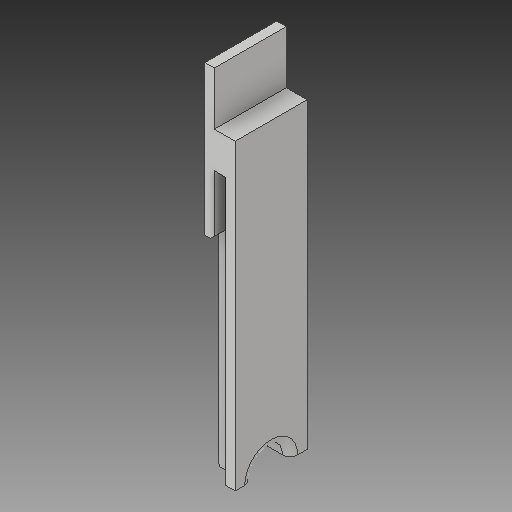
# Autodesk Inventor part: BOttom Clip
Saved by Autodesk Inventor 2017 (Build 210142000, 142)
## iProperties
Created: 2018-02-13
Part Number: BOttom Clip
Material: Generic
Document SubType Name: Modeling
Designer: Arjuna
Density: 1 g/cm^3
Appearance: Default
Author: Arjuna
Autodesk Inventor part; units mm, degrees
ref_plane "YZ Plane" through (0, 0, 0) normal (1, 0, 0) x (0, 1, 0)
ref_plane "XZ Plane" through (0, 0, 0) normal (0, 1, 0) x (-1, 0, 0)
ref_plane "XY Plane" through (0, 0, 0) normal (0, 0, 1) x (1, 0, 0)
sketch "Sketch1" plane through (0, 0, 0) normal (1, 0, 0) x (0, 1, 0)
  line L0 (40, 9.5) -> (-40, 9.5)
  line L1 (-40, 9.5) -> (-40, -9.5)
  line L2 (-40, -9.5) -> (40, -9.5)
  line L3 (40, -9.5) -> (40, 9.5)
  point P0 (0, 0)
  dimension "d0" = 19
  dimension "d1" = 80
  dimension "d2" = 9.5
  dimension "d3" = 40
  constraints: 8 end point, 2 parallel, 1 horizontal, 1 perpendicular
  measures "d0" distance between parallel lines of L2 L0
  measures "d1" distance between parallel lines of L1 L3
  measures "d2" distance from line of L0 point (0, 0)
  measures "d3" distance from line of point (0, 0) L3
extrude "Extrusion1" add sketch "Sketch1" along normal blind 8
sketch "Sketch2" plane through (0, 40, 9.5) normal (0, 1, 0) x (1, 0, 0)
  line L0 (0, 19) -> (0, 0) projected
  line L1 (0, 0) -> (8, 0) projected
  line L2 (8, 19) -> (8, 0) projected
  line L3 (0, 19) -> (8, 19) projected
  line L4 (0, 0) -> (2.5, 0)
  line L5 (2.5, 0) -> (2.5, 19)
  line L6 (2.5, 19) -> (0, 19)
  line L7 (0, 19) -> (0, 0)
  point P0 (0, 9.5)
  dimension "d6" = 2.5
  constraints: 8 end point, 2 parallel, 1 horizontal, 1 perpendicular, 1 point on line
  measures "d6" distance of L6.end L5.end
extrude "Extrusion2" add sketch "Sketch2" along normal blind 14 contours L3 L5 L1 L0
sketch "Sketch4" plane through (8, -40, -9.5) normal (0, 0, -1) x (-1, 0, 0)
  line L0 (8, 0) -> (8, 94) projected
  line L1 (5.5, 94) -> (8, 94) projected
  line L2 (5.5, 80) -> (5.5, 94) projected
  line L3 (5.5, 80) -> (0, 80) projected
  line L4 (0, 0) -> (0, 80) projected
  line L5 (8, 0) -> (0, 0) projected
  line L6 (2.5, 70.5) -> (5.5, 70.5)
  line L7 (5.5, 70.5) -> (5.5, 54.5)
  line L8 (5.5, 54.5) -> (2.5, 54.5)
  line L9 (2.5, 54.5) -> (2.5, 70.5)
  line L10 (2.5, 54.5) -> (8, 54.5)
  line L11 (8, 54.5) -> (8, 0)
  line L12 (8, 0) -> (2.5, 0)
  line L13 (2.5, 0) -> (2.5, 54.5)
  point P0 (8, 40)
  dimension "d9" = 3
  dimension "d10" = 9.5
  dimension "d11" = 16
  dimension "d12" = 2.5
  dimension "d13" = 2.5
  constraints: 16 end point, 4 parallel, 2 horizontal, 2 perpendicular
  measures "d9" distance of L7.end L8.end
  measures "d10" distance between parallel lines of L6 L3
  measures "d11" distance between parallel lines of L8 L6
  measures "d12" distance between parallel lines of L9 L4
  measures "d13" distance between parallel lines of L0 L7
extrude "Extrusion3" cut sketch "Sketch4" against normal blind 3.5 contours L5 L13 L8 L10 L0 | L8 L9 L6 L7
mirror "Mirror1" about plane through (0, 0, 0) normal (0, 0, 1) of "Extrusion3"
chamfer "Chamfer1" distance 1 angle 45 2 edges at (2.5, 14.5, 7.75) (2.5, 14.5, -7.75)
sketch "Sketch5" plane through (8, 0, 0) normal (1, 0, 0) x (0, 0, -1)
  line L0 (-9.5, 40) -> (-9.5, -40) projected
  line L1 (-9.5, -40) -> (9.5, -40) projected
  line L2 (9.5, -40) -> (9.5, 40) projected
  line L3 (9.5, 40) -> (-9.5, 40) projected
  circle A0 centre (0, -40) radius 5
  point P0 (0, 0)
  dimension "d19" = 10
  constraints: 1 centre point, 1 midpoint
  measures "d19" diameter of A0
extrude "Extrusion4" cut sketch "Sketch5" against normal through all contours A0 L1 | L1 A0
fillet "Fillet1" radius 2 2 edges at (8, -35, 0) (0, -35, 0)
equation "\"d2\" = 0.5 * d0"
equation "\"d3\" = 0.5 * d1"
body "Solid1"
